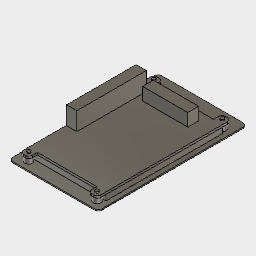
2441 PiTFT 3.5 (Autodesk Fusion 360 design; units mm, degrees)
Autodesk Fusion 360 part; units mm, degrees
sketch "PCB" plane through (0, 0, 0) normal (0, 0, 1) x (1, 0, 0)
  line L0 (0, 0) -> (56.52, 0)
  line L1 (56.52, 0) -> (56.52, 84.96)
  line L2 (56.52, 84.96) -> (0, 84.96)
  line L3 (0, 84.96) -> (0, 0)
  line L4 (0, 84.96) -> (6.6, 84.96)
  line L5 (6.6, 84.96) -> (6.6, 91.16)
  line L6 (6.6, 91.16) -> (0, 91.16)
  line L7 (0, 91.16) -> (0, 84.96)
  line L8 (3.3, 91.16) -> (3.3, 84.96) construction
  line L9 (0, 88.06) -> (6.6, 88.06) construction
  circle A0 centre (3.3, 88.06) radius 1.25
  line L10 (28.26, 84.96) -> (28.26, 0) construction
  line L11 (0, 42.48) -> (56.52, 42.48) construction
  circle A1 centre (53.22, 88.06) radius 1.25
  line L12 (49.92, 91.16) -> (56.52, 91.16)
  line L13 (56.52, 91.16) -> (56.52, 84.96)
  line L14 (49.92, 84.96) -> (49.92, 91.16)
  line L15 (0, -6.2) -> (0, 0)
  line L16 (6.6, -6.2) -> (0, -6.2)
  circle A2 centre (3.3, -3.1) radius 1.25
  line L17 (6.6, 0) -> (6.6, -6.2)
  circle A3 centre (53.22, -3.1) radius 1.25
  line L18 (49.92, -6.2) -> (56.52, -6.2)
  line L19 (49.92, 0) -> (49.92, -6.2)
  line L20 (56.52, -6.2) -> (56.52, 0)
  dimension "d1" = 84.96
  dimension "d2" = 56.52
  dimension "d3" = 6.6
  dimension "d4" = 6.2
  dimension "d5" = 2.5
  dimension "d6" = 49.92
  dimension "d7" = 91.16
  measures "d1" distance of L0.start L2.end
  measures "d2" distance of L0.start L0.end
  measures "d3" distance of L2.end L4.end
  measures "d4" distance of L2.end L6.end
  measures "d5" diameter of A0
  measures "d6" distance of A0.centre A1.centre
  measures "d7" distance of A1.centre A3.centre
extrude "Extrude1" add sketch "PCB" against normal blind 1.6 makes body 1
fillet "Fillet1" radius 2.54 8 edges at (0, -6.2, -0.8) (6.6, -6.2, -0.8) (49.92, -6.2, -0.8) (56.52, -6.2, -0.8) (49.92, 91.16, -0.8) (56.52, 91.16, -0.8) (6.6, 91.16, -0.8) (0, 91.16, -0.8) on bodies 1
sketch "headers" plane through (0, 0, 0) normal (0, 0, 1) x (1, 0, 0)
  line L0 (0, 0) -> (56.52, 0)
  line L1 (56.52, 0) -> (56.52, 84.96)
  line L2 (56.52, 84.96) -> (0, 84.96)
  line L3 (0, 84.96) -> (0, 0)
  line L4 (45.46, 70.735) -> (12.46, 70.735)
  line L5 (12.46, 70.735) -> (12.46, 78.605)
  line L6 (12.46, 78.605) -> (45.46, 78.605)
  line L7 (45.46, 78.605) -> (45.46, 70.735)
  line L8 (45.46, 70.735) -> (12.46, 78.605) construction
  line L9 (12.46, 70.735) -> (45.46, 78.605) construction
  line L10 (0.254, 78.23) -> (7.874, 78.23)
  line L11 (7.874, 78.23) -> (7.874, 27.43)
  line L12 (7.874, 27.43) -> (0.254, 27.43)
  line L13 (0.254, 27.43) -> (0.254, 78.23)
  point P0 (28.96, 74.67)
  dimension "d11" = 84.96
  dimension "d12" = 56.52
  dimension "d13" = 33
  dimension "d14" = 7.87
  dimension "d15" = 28.96
  dimension "d16" = 10.29
  dimension "d17" = 7.62
  dimension "d18" = 50.8
  dimension "d19" = 6.73
  dimension "d20" = 0.254
  measures "d11" distance of L0.start L2.end
  measures "d12" distance of L0.start L0.end
  measures "d13" distance of L5.end L6.end
  measures "d14" distance of L4.end L5.end
  measures "d15" distance of L3 P0
  measures "d16" distance of L2 P0
  measures "d17" distance of L10.start L10.end
  measures "d18" distance of L10.start L12.end
  measures "d19" distance of L2 L10
  measures "d20" distance of L3 L13
extrude "Extrude2" add sketch "headers" along normal blind 9.2 contours L4 L5 L6 L7 bodies 1
extrude "Extrude3" add sketch "headers" along normal blind 13.2 contours L10 L11 L12 L13 bodies 1
sketch "screen cut" plane through (0, 0, -1.6) normal (0, 0, -1) x (1, 0, 0)
  line L0 (0, 0) -> (56.52, 0)
  line L1 (56.52, 0) -> (56.52, -84.96)
  line L2 (56.52, -84.96) -> (0, -84.96)
  line L3 (0, -84.96) -> (0, 0)
  line L4 (53.02, -82.96) -> (2, -82.96)
  line L5 (2, -82.96) -> (2, -7.2)
  line L6 (2, -7.2) -> (53.02, -7.2)
  line L7 (53.02, -7.2) -> (53.02, -82.96)
  dimension "d48" = 84.96
  dimension "d49" = 56.52
  dimension "d50" = 7.2
  dimension "d51" = 3.5
  dimension "d52" = 2
  dimension "d53" = 2
  measures "d48" distance of L0.start L2.end
  measures "d49" distance of L0.start L0.end
  measures "d50" distance of L0 L6
  measures "d51" distance of L1 L7
  measures "d52" distance of L2 L4
  measures "d53" distance of L3 L5
extrude "Extrude4" add sketch "screen cut" along normal blind 4 separate body contours L0 L1 L2 L3 | L4 L5 L6 L7 makes body 2
sketch "display mount" plane through (0, 0, -5.6) normal (0, 0, -1) x (1, 0, 0)
  line L0 (0, -84.96) -> (56.52, -84.96) construction
  line L1 (56.52, -84.96) -> (56.52, 0) construction
  line L2 (56.52, 0) -> (0, 0) construction
  line L3 (0, 0) -> (0, -84.96) construction
  line L4 (-5, 9.2) -> (60.02, 9.2)
  line L5 (60.02, 9.2) -> (60.02, -99.36)
  line L6 (60.02, -99.36) -> (-5, -99.36)
  line L7 (-5, -99.36) -> (-5, 9.2)
  circle A0 centre (3.3, -88.06) radius 1.25
  circle A1 centre (53.22, -88.06) radius 1.25
  circle A2 centre (53.22, 3.1) radius 1.25
  circle A3 centre (3.3, 3.1) radius 1.25
  circle A4 centre (3.3, -88.06) radius 2.75
  circle A5 centre (53.22, 3.1) radius 2.75
  circle A6 centre (3.3, 3.1) radius 2.75
  circle A7 centre (53.22, -88.06) radius 2.75
  line L8 (56.52, 3.66) -> (56.52, -88.62)
  line L9 (0, -88.62) -> (0, 3.66)
  line L10 (4.06, -91.16) -> (2.54, -91.16)
  line L11 (4.06, 6.2) -> (2.54, 6.2)
  dimension "d54" = 5.5
  dimension "d55" = 5.5
  dimension "d56" = 5.5
  dimension "d57" = 5.5
  dimension "d64" = 3.5
  dimension "d65" = 5
  dimension "d66" = 8.2
  dimension "d67" = 3
  measures "d54" diameter of A4
  measures "d55" diameter of A5
  measures "d56" diameter of A6
  measures "d57" diameter of A7
  measures "d64" distance of L5 L8
  measures "d65" distance of L7 L9
  measures "d66" distance of L6 L10
  measures "d67" distance of L4 L11
extrude "Extrude9" add sketch "display mount" along normal blind 1 separate body contours L4 L5 L6 L7 | A0 | A1 | A2 | A3 | A4 | A5 | A6 | A7 makes body 3
extrude "Extrude10" cut sketch "screen cut" along normal up to surface (5 mm away) contours L4 L5 L6 L7 bodies 3
extrude "Extrude11" add sketch "display mount" against normal up to surface (4 mm away) contours A0 | A1 | A2 | A3 | A4 | A5 | A6 | A7 bodies 3
extrude "Extrude12" add sketch "display mount" against normal blind 6.5 contours A0 | A1 | A2 | A3 bodies 3
fillet "Fillet3" radius 3 4 edges at (60.02, -9.2, -6.1) (-5, -9.2, -6.1) (-5, 99.36, -6.1) (60.02, 99.36, -6.1) on bodies 3
named bodies: "PCB", "display", "mount"
